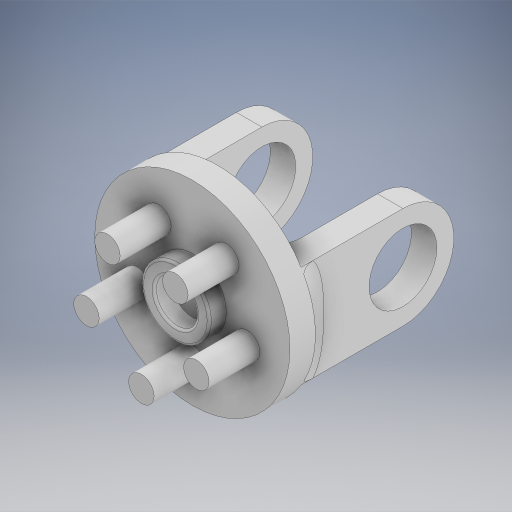
# Autodesk Inventor part: wheel hub
Saved by Autodesk Inventor 2024 (Build 280153000, 153)
## iProperties
Created: 2024-04-03
Part Number: wheel hub
Material: Generic
Document SubType Name: Modeling
Designer: Alex
Density: 1 g/cm^3
Appearance: Default
Author: Alex
Autodesk Inventor part; units mm, degrees
ref_plane "YZ Plane" through (0, 0, 0) normal (1, 0, 0) x (0, 1, 0)
ref_plane "XZ Plane" through (0, 0, 0) normal (0, 1, 0) x (-1, 0, 0)
ref_plane "XY Plane" through (0, 0, 0) normal (0, 0, 1) x (1, 0, 0)
sketch "Sketch1" plane through (0, 0, 0) normal (0, 0, 1) x (1, 0, 0)
  line L0 (0, -6.8052) -> (-6.4721, -2.1029) construction
  line L1 (-6.4721, -2.1029) -> (-4, 5.5055) construction
  line L2 (-4, 5.5055) -> (4, 5.5055) construction
  line L3 (4, 5.5055) -> (6.4721, -2.1029) construction
  line L4 (6.4721, -2.1029) -> (0, -6.8052) construction
  circle A0 centre (4, 5.5055) radius 1.5
  circle A1 centre (6.4721, -2.1029) radius 1.5
  circle A2 centre (0, -6.8052) radius 1.5
  circle A3 centre (-6.4721, -2.1029) radius 1.5
  circle A4 centre (-4, 5.5055) radius 1.5
  line L5 (0, -6.8052) -> (0, 5.5055) construction
  circle A5 centre (0, 0) radius 11.5
  circle A6 centre (0, 0) radius 4
  circle A7 centre (0, 0) radius 2.5
  dimension "d0" = 8
  dimension "d1" = 3
  dimension "d2" = 3
  dimension "d3" = 3
  dimension "d4" = 3
  dimension "d5" = 3
  dimension "d6" = 23
  dimension "d7" = 8
  dimension "d8" = 1.5
  constraints: 12 end point, 8 centre point, 8 coincident, 1 midpoint, 1 vertical, 11 other
  measures "d0" distance of L1.end L2.end
  measures "d1" diameter of A0
  measures "d2" diameter of A1
  measures "d3" diameter of A2
  measures "d4" diameter of A3
  measures "d5" diameter of A4
  measures "d6" diameter of A5
  measures "d7" diameter of A6
  measures "d8" radial gap between concentric circles of A6 A7
extrude "Extrusion1" add sketch "Sketch1" against normal blind 3 contours A0 | A1 | A2 | A3 | A4 | A5 | A6 | A7
extrude "Extrusion2" add sketch "Sketch1" along normal blind 2 contours A6
fillet "Fillet1" radius 0.25 1 edges at (-4, 0, 2)
fillet "Fillet2" radius 0.25 1 edges at (-2.5, 0, 2)
extrude "Extrusion3" add sketch "Sketch1" along normal blind 6 contours A0 | A1 | A2 | A3 | A4
sketch "Sketch2" plane through (0, 0, -3) normal (0, 0, -1) x (-1, 0, 0)
  line L0 (-9.8107, 6) -> (-6.8107, 6)
  line L1 (-6.8107, 6) -> (-6.8107, -6)
  line L2 (-6.8107, -6) -> (-9.8107, -6)
  line L3 (-9.8107, -6) -> (-9.8107, 6)
  line L4 (6.8107, 6) -> (9.8107, 6)
  line L5 (9.8107, 6) -> (9.8107, -6)
  line L6 (9.8107, -6) -> (6.8107, -6)
  line L7 (6.8107, -6) -> (6.8107, 6)
  circle A0 centre (0, 0) radius 11.5 construction
  line L8 (0, 11.5) -> (0, -11.5) construction
  point P0 (6.8107, 0)
  dimension "d18" = 3
  dimension "d19" = 12
  constraints: 18 end point, 4 parallel, 3 point on circle, 2 equal length, 2 horizontal, 2 horizontal alignment, 2 midpoint, 2 perpendicular, 1 coincident, 1 point on line, 1 vertical, 1 other
  measures "d18" distance of L4.start L4.end
  measures "d19" distance of L4.end L5.end
extrude "Extrusion4" add sketch "Sketch2" along normal blind 18
fillet "Fillet3" radius 6 4 edges at (8.3107, 6, -21) (8.3107, -6, -21) (-8.3107, 6, -21) (-8.3107, -6, -21)
sketch "Sketch3" plane through (9.8107, -6, -3) normal (1, 0, 0) x (0, 0, -1)
  arc A0 (12, 0) -> (12, 12) centre (12, 6) ccw construction
  circle A1 centre (12, 6) radius 4
  point P0 (-3, 6)
  dimension "d23" = 8
  constraints: 1 centre point, 1 coincident
  measures "d23" diameter of A1
extrude "Extrusion5" cut sketch "Sketch3" against normal through all
fillet "Fillet4" radius 3 2 edges at (6.8107, 0, -3) (-6.8107, 0, -3)
fillet "Fillet5" radius 3 2 edges at (9.8107, 0, -3) (-9.8107, 0, -3)
equation "\"d2\" = d1"
equation "\"d3\" = d1"
equation "\"d4\" = d1"
equation "\"d5\" = d1"
body "Solid1"
